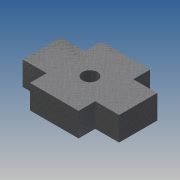
# Autodesk Inventor part: Kugellager-Schieber-Druckplatte
Saved by Autodesk Inventor 2015 SP1 (Build 190203100, 203)
## iProperties
Created: 2015-01-28
Part Number: Kugellager-Schieber-Druckplatte
Material: ABS-Kunststoff
Document SubType Name: Modeling
Designer: Marc
Mass: 1.16801 g
Surface Area: 8.45736 cm^2
Volume: 1.10189 cm^3
Density: 1.06 g/cm^3
Appearance: Gehont - dunkelgrau
Author: Marc
Autodesk Inventor part; units mm, degrees
ref_plane "YZ Plane" through (0, 0, 0) normal (1, 0, 0) x (0, 1, 0)
ref_plane "XZ Plane" through (0, 0, 0) normal (0, 1, 0) x (-1, 0, 0)
ref_plane "XY Plane" through (0, 0, 0) normal (0, 0, 1) x (1, 0, 0)
sketch "Skizze1" plane through (0, 0, 0) normal (0, 0, 1) x (1, 0, 0)
  line L0 (0, -10.5) -> (0, 10.5) projected
  line L1 (-14.14, 0) -> (14.14, 0) projected
  line L2 (-5.1, -7.5) -> (5.1, -7.5)
  line L3 (5.1, -7.5) -> (5.1, 7.5)
  line L4 (5.1, 7.5) -> (-5.1, 7.5)
  line L5 (-5.1, 7.5) -> (-5.1, -7.5)
  line L6 (-5.1, 4) -> (-10.1, 4)
  line L7 (-10.1, 4) -> (-10.1, -4)
  line L8 (-10.1, -4) -> (-5.1, -4)
  line L9 (-5.1, -4) -> (-5.1, 4)
  line L10 (5.1, 4) -> (10.1, 4)
  line L11 (10.1, 4) -> (10.1, -4)
  line L12 (10.1, -4) -> (5.1, -4)
  line L13 (5.1, -4) -> (5.1, 4)
  circle A0 centre (0, 0) radius 1.55
  dimension "d0" = 10.2
  dimension "d1" = 15
  dimension "d2" = 5
  dimension "d3" = 8
  dimension "d4" = 3.1
  constraints: 24 end point, 4 parallel, 4 symmetric about line, 2 horizontal, 2 perpendicular, 1 centre point, 1 coincident, 1 point on line, 3 other
  measures "d0" distance of L4.end L3.end
  measures "d1" distance of L3.end L2.end
  measures "d2" distance of L8.end L7.end
  measures "d3" distance of L7.end L6.end
  measures "d4" diameter of A0
extrude "Extrusion1" add sketch "Skizze1" along normal blind 5 contours L2 L5 L1 A0 L0 | L0 A0 L1 L3 L2 | L1 L5 L4 L0 A0 | A0 L0 L4 L3 L1 | L8 L7 L1 L5 | L3 L1 L11 L12 | L1 L7 L6 L5 | L3 L10 L11 L1
